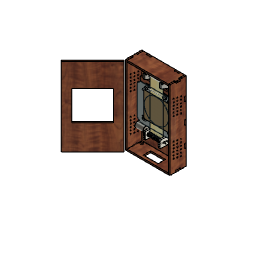
Target Holder v0 (Autodesk Fusion 360 design; units mm, degrees)
Autodesk Fusion 360 part; units mm, degrees
note: some values were not read from the file. Set by a fixed rule: which face or edge a step refers to.
(part 1 of 4)
sketch "Sketch8" plane through (0, 0, 0) normal (0, 1, 0) x (1, 0, 0)
  line L0 (-142.6941, 256.8986) -> (-422.6941, 256.8986)
  line L1 (-232.6941, -163.1014) -> (-332.6941, -163.1014)
  line L2 (-365.1941, -98.1014) -> (-200.1941, -98.1014)
  line L3 (-200.1941, -98.1014) -> (-200.1941, 66.8986)
  line L4 (-200.1941, 66.8986) -> (-365.1941, 66.8986)
  line L5 (-365.1941, 66.8986) -> (-365.1941, -98.1014)
  line L6 (-392.6941, -273.1014) -> (-362.6941, -273.1014)
  line L7 (-362.6941, -273.1014) -> (-362.6941, -263.1014)
  line L8 (-392.6941, -263.1014) -> (-392.6941, -273.1014)
  line L9 (-432.6941, -18.1014) -> (-422.6941, -18.1014)
  line L10 (-422.6941, 11.8986) -> (-432.6941, 11.8986)
  line L11 (-432.6941, 11.8986) -> (-432.6941, -18.1014)
  line L12 (-142.6941, -18.1014) -> (-132.6941, -18.1014)
  line L13 (-132.6941, -18.1014) -> (-132.6941, 11.8986)
  line L14 (-132.6941, 11.8986) -> (-142.6941, 11.8986)
  line L15 (-432.6941, -155.6014) -> (-422.6941, -155.6014)
  line L16 (-422.6941, -125.6014) -> (-432.6941, -125.6014)
  line L17 (-432.6941, -125.6014) -> (-432.6941, -155.6014)
  line L18 (-142.6941, 119.3986) -> (-132.6941, 119.3986)
  line L19 (-132.6941, 119.3986) -> (-132.6941, 149.3986)
  line L20 (-132.6941, 149.3986) -> (-142.6941, 149.3986)
  line L21 (-142.6941, -140.6014) -> (-132.6941, -140.6014)
  line L22 (-132.6941, -140.6014) -> (-132.6941, -110.6014)
  line L23 (-132.6941, -110.6014) -> (-142.6941, -110.6014)
  line L24 (-432.6941, 119.3986) -> (-422.6941, 119.3986)
  line L25 (-422.6941, 149.3986) -> (-432.6941, 149.3986)
  line L26 (-432.6941, 149.3986) -> (-432.6941, 119.3986)
  line L27 (-422.6941, -23.1014) -> (-422.6941, -120.6038)
  line L28 (-422.6941, -155.6014) -> (-422.6941, -263.1014)
  line L29 (-422.6941, 256.8986) -> (-422.6941, 154.3986)
  line L30 (-422.6941, 114.3986) -> (-422.6941, 16.8986)
  line L31 (-142.6941, 16.8986) -> (-142.6941, 114.3986)
  line L32 (-142.6941, 149.3986) -> (-142.6941, 256.8986)
  line L33 (-142.6941, -263.1014) -> (-142.6941, -145.6014)
  line L34 (-142.6941, -105.6014) -> (-142.6941, -23.1014)
  line L35 (-422.6941, -263.1014) -> (-397.6941, -263.1014)
  line L36 (-357.6941, -263.1014) -> (-332.6941, -263.1014)
  arc A0 (-422.6941, -160.6014) -> (-422.6941, -155.6014) centre (-422.6941, -158.1014) ccw
  arc A1 (-422.8505, -125.6014) -> (-422.6941, -120.6038) centre (-422.7723, -123.1026) ccw
  arc A2 (-422.6941, -23.1014) -> (-422.6941, -18.1014) centre (-422.6941, -20.6014) ccw
  arc A3 (-422.6941, 11.8986) -> (-422.6941, 16.8986) centre (-422.6941, 14.3986) ccw
  arc A4 (-142.6941, -18.1014) -> (-142.6941, -23.1014) centre (-142.6941, -20.6014) ccw
  arc A5 (-142.6941, 16.8986) -> (-142.6941, 11.8986) centre (-142.6941, 14.3986) ccw
  arc A6 (-142.6941, -140.6014) -> (-142.6941, -145.6014) centre (-142.6941, -143.1014) ccw
  arc A7 (-142.6941, -105.6014) -> (-142.6941, -110.6014) centre (-142.6941, -108.1014) ccw
  arc A8 (-392.6941, -263.1014) -> (-397.6941, -263.1014) centre (-395.1941, -263.1014) ccw
  arc A9 (-357.6941, -263.1014) -> (-362.6941, -263.1014) centre (-360.1941, -263.1014) ccw
  line L37 (-202.6941, -273.1014) -> (-172.6941, -273.1014)
  line L38 (-172.6941, -273.1014) -> (-172.6941, -263.1014)
  line L39 (-202.6941, -263.1014) -> (-202.6941, -273.1014)
  arc A10 (-202.6941, -263.1014) -> (-207.6941, -263.1014) centre (-205.1941, -263.1014) ccw
  line L40 (-232.6941, -263.1014) -> (-207.6941, -263.1014)
  line L41 (-167.6941, -263.1014) -> (-142.6941, -263.1014)
  arc A11 (-167.6941, -263.1014) -> (-172.6941, -263.1014) centre (-170.1941, -263.1014) ccw
  arc A12 (-422.6941, 114.3986) -> (-422.6941, 119.3986) centre (-422.6941, 116.8986) ccw
  arc A13 (-422.6941, 149.3986) -> (-422.6941, 154.3986) centre (-422.6941, 151.8986) ccw
  arc A14 (-142.6941, 119.3986) -> (-142.6941, 114.3986) centre (-142.6941, 116.8986) ccw
  arc A15 (-142.6941, 154.3986) -> (-142.6941, 149.3986) centre (-142.6941, 151.8986) ccw
  line L42 (-332.6941, -163.1014) -> (-232.6941, -163.1014)
  line L43 (-232.6941, -213.1014) -> (-332.6941, -213.1014)
  line L44 (-232.6941, -198.1014) -> (-232.6941, -200.1678)
  line L45 (-342.6941, -198.1014) -> (-332.6941, -198.1014)
  line L46 (-332.6941, -178.1014) -> (-342.6941, -178.1014)
  line L47 (-342.6941, -183.1014) -> (-342.6941, -193.1014)
  line L48 (-332.6941, -163.1014) -> (-332.6941, -178.1014)
  line L49 (-332.6941, -198.1014) -> (-332.6941, -263.1014)
  line L50 (-332.6941, -213.1014) -> (-332.6941, -198.1014)
  line L51 (-332.6941, -178.1014) -> (-332.6941, -163.1014)
  line L52 (-232.6941, -198.1014) -> (-222.6941, -198.1014)
  line L53 (-222.6941, -178.1014) -> (-232.6941, -178.1014)
  line L54 (-232.6941, -263.1014) -> (-232.6941, -198.1014)
  line L55 (-232.6941, -178.1014) -> (-232.6941, -163.1014)
  line L56 (-232.6941, -163.1014) -> (-232.6941, -178.1014)
  line L57 (-232.6941, -198.1014) -> (-232.6941, -213.1014)
  arc A16 (-222.6941, -198.1014) -> (-222.6941, -193.1014) centre (-222.6941, -195.6014) ccw
  arc A17 (-222.6941, -183.1014) -> (-222.6941, -178.1014) centre (-222.6941, -180.6014) ccw
  arc A18 (-342.6941, -193.1014) -> (-342.6941, -198.1014) centre (-342.6941, -195.6014) ccw
  arc A19 (-342.6941, -178.1014) -> (-342.6941, -183.1014) centre (-342.6941, -180.6014) ccw
  line L58 (-222.6941, -193.1014) -> (-222.6941, -183.1014)
  dimension "d24" = 280
  dimension "d25" = 520
  dimension "d26" = 100
  dimension "d27" = 100
  dimension "d28" = 165
  dimension "d29" = 165
  dimension "d36" = 30
  dimension "d37" = 10
  dimension "d40" = 10
  dimension "d41" = 30
  dimension "d42" = 10
  dimension "d43" = 30
  dimension "d44" = 10
  dimension "d45" = 30
  dimension "d46" = 10
  dimension "d47" = 30
  dimension "d48" = 10
  dimension "d49" = 30
  dimension "d50" = 10
  dimension "d51" = 30
  dimension "d52" = 5
  dimension "d53" = 5
  dimension "d54" = 5
  dimension "d55" = 5
  dimension "d56" = 5
  dimension "d57" = 5
  dimension "d58" = 5
  dimension "d59" = 5
  dimension "d60" = 5
  dimension "d61" = 5
  dimension "d63" = 30
  dimension "d64" = 10
  dimension "d65" = 5
  dimension "d66" = 5
  dimension "d67" = 5
  dimension "d68" = 5
  dimension "d69" = 5
  dimension "d70" = 5
  dimension "d73" = 50
  dimension "d76" = 10
  dimension "d77" = 20
  dimension "d78" = 10
  dimension "d79" = 20
  dimension "d80" = 5
  dimension "d81" = 5
  dimension "d82" = 5
  dimension "d84" = 5
  constraint horizontal L35
  constraint vertical L33
  constraint horizontal L0
  constraint vertical L29
  constraint vertical L54
  constraint horizontal L1
  constraint vertical L48
  constraint horizontal L2
  constraint vertical L3
  constraint horizontal L4
  constraint vertical L5
  constraint horizontal L6
  constraint vertical L7
  constraint vertical L8
  constraint horizontal L9
  constraint horizontal L10
  constraint vertical L11
  constraint horizontal L12
  constraint vertical L13
  constraint horizontal L14
  constraint horizontal L15
  constraint horizontal L16
  constraint vertical L17
  constraint horizontal L18
  constraint vertical L19
  constraint horizontal L20
  constraint horizontal L21
  constraint vertical L22
  constraint horizontal L23
  constraint collinear L31 L33
  constraint collinear L27 L29
  constraint horizontal L24
  constraint horizontal L25
  constraint vertical L26
  constraint collinear L27 L28
  constraint collinear L29 L30
  constraint collinear L31 L32
  constraint collinear L33 L34
  constraint collinear L35 L36
  constraint coincident L16.start A1
  constraint coincident L28 A0.start
  constraint coincident L16 A1.start
  constraint perpendicular L33 L40
  constraint horizontal L37
  constraint vertical L38
  constraint vertical L39
  constraint collinear L40 L41
  constraint coincident L32 A15.start
  constraint horizontal L42
  constraint vertical L56
  constraint horizontal L43
  constraint vertical L50
  constraint vertical L44
  constraint coincident L44.end L54
  constraint coincident L44.end L56
  constraint horizontal L45
  constraint horizontal L46
  constraint vertical L47
  constraint collinear L48 L49
  constraint collinear L50 L51
  constraint horizontal L52
  constraint horizontal L53
  constraint collinear L54 L55
  constraint collinear L56 L57
  constraint vertical L58
  measures "d24" distance of L28.end L33.start
  measures "d25" distance of L28.end L0.end
  measures "d26" distance of L36.end L40.start
  measures "d27" distance of L36.end L1.end
  measures "d28" distance of L2.start L2.end
  measures "d29" distance of L2.start L4.end
  measures "d36" distance of L6.start L6.end
  measures "d37" distance of L6.start L8.start
  measures "d40" distance of L9.start L9.end
  measures "d41" distance of L9.start L10.end
  measures "d42" distance of L12.start L12.end
  measures "d43" distance of L12.start L14.end
  measures "d44" distance of L15.start L15.end
  measures "d45" distance of L15.start L16.end
  measures "d46" distance of L18.start L18.end
  measures "d47" distance of L18.start L20.end
  measures "d48" distance of L21.start L21.end
  measures "d49" distance of L21.start L23.end
  measures "d50" distance of L24.start L24.end
  measures "d51" distance of L24.start L25.end
  measures "d52" diameter of A0
  measures "d53" diameter of A1
  measures "d54" diameter of A2
  measures "d55" diameter of A3
  measures "d56" diameter of A4
  measures "d57" diameter of A5
  measures "d58" diameter of A6
  measures "d59" diameter of A7
  measures "d60" diameter of A8
  measures "d61" diameter of A9
  measures "d63" distance of L37.start L37.end
  measures "d64" distance of L37.start L39.start
  measures "d65" diameter of A10
  measures "d66" diameter of A11
  measures "d67" diameter of A12
  measures "d68" diameter of A13
  measures "d69" diameter of A15
  measures "d70" diameter of A14
  measures "d73" distance of L1.end L43.end
  measures "d76" distance of L45.start L45.end
  measures "d77" distance of L45.start L46.end
  measures "d78" distance of L44.start L52.end
  measures "d79" distance of L44.start L53.end
  measures "d80" diameter of A17
  measures "d81" diameter of A16
  measures "d82" diameter of A19
  measures "d84" diameter of A18
sketch "Sketch9" plane through (0, 0, 0) normal (0, 1, 0) x (1, 0, 0)
extrude "Extrude1" add sketch "Sketch8" along normal blind 10 contours L0 L1 L6 L7 L8 L9 L10 L11 L12 L13 L14 L15 L16 L17 L18 L19 L20 L21 L22 L23 L24 L25 L26 L27 L28 L29 L30 L31 L32 L33 L34 L35 L36 A0 A1 A2 A3 A4 A5 A6 A7 A8 A9 L37 L38 L39 A10 L40 L41 A11 A12 A13 A14 A15 L42 L44 L45 L46 L47 L48 L49 L50 L51 L52 L53 L54 L55 L56 L57 A16 A17 A18 A19 L58 makes body 1
sketch "Sketch1" plane through (0, 0, 0) normal (1, 0, 0) x (0, 1, 0) in component "Side"
sketch "Sketch2" plane through (-142.6941, 0, 0) normal (1, 0, 0) x (0, 1, 0) in component "Side"
sketch "Sketch3" plane through (0, 0, 0) normal (0, -1, 0) x (1, 0, 0) in component "Side"
sketch "Sketch10" plane through (-142.6941, 0, 0) normal (1, 0, 0) x (0, 1, 0)
  line L0 (-100, -256.3488) -> (-100, 273.6512)
  line L1 (0, -119.3986) -> (10, -119.3986)
  line L2 (10, -149.3986) -> (0, -149.3986)
  line L3 (0, -144.3986) -> (0, -124.3986)
  line L4 (0, 140.6014) -> (10, 140.6014)
  line L5 (10, 110.6014) -> (0, 110.6014)
  line L6 (0, 110.6014) -> (0, 115.6014)
  line L7 (0, 18.1014) -> (10, 18.1014)
  line L8 (10, -11.8986) -> (0, -11.8986)
  line L9 (0, -6.8986) -> (0, 13.1014)
  line L10 (10, 273.6512) -> (10, 140.6014)
  arc A0 (0, 140.6014) -> (0, 135.6014) centre (0, 138.1014) ccw
  arc A1 (0, 115.6014) -> (0, 110.6014) centre (0, 113.1014) ccw
  line L11 (10, 110.6014) -> (10, 18.1014)
  arc A2 (0, -6.8986) -> (0, -11.8986) centre (0, -9.3986) ccw
  arc A3 (0, 18.1014) -> (0, 13.1014) centre (0, 15.6014) ccw
  arc A4 (0, -119.3986) -> (0, -124.3986) centre (0, -121.8986) ccw
  arc A5 (0, -144.3986) -> (0, -149.3986) centre (0, -146.8986) ccw
  line L12 (-30, 273.6512) -> (-30, 263.6512)
  line L13 (-35, 263.6512) -> (-55, 263.6512)
  line L14 (-60, 263.6512) -> (-60, 273.6512)
  line L15 (-100, 273.6512) -> (-60, 273.6512)
  line L16 (-30, 273.6512) -> (10, 273.6512)
  arc A6 (-60, 263.6512) -> (-55, 263.6512) centre (-57.5, 263.6512) ccw
  arc A7 (-35, 263.6512) -> (-30, 263.6512) centre (-32.5, 263.6512) ccw
  circle A8 centre (-75, 230) radius 4
  circle A9 centre (-55, 225) radius 4
  circle A10 centre (-35, 220) radius 4
  line L17 (-55, -246.3488) -> (-35, -246.3488)
  line L18 (-30, -246.3488) -> (-30, -256.3488)
  line L19 (-60, -256.3488) -> (-60, -246.3488)
  line L20 (10, -256.3488) -> (-30, -256.3488)
  line L21 (-60, -256.3488) -> (-100, -256.3488)
  arc A11 (-55, -246.3488) -> (-60, -246.3488) centre (-57.5, -246.3488) ccw
  arc A12 (-30, -246.3488) -> (-35, -246.3488) centre (-32.5, -246.3488) ccw
  line L22 (10, -11.8986) -> (10, -119.3986)
  line L23 (10, -149.3986) -> (10, -256.3488)
  line L24 (0, 135.6014) -> (0, 115.6014)
  point P0 (0, -256.8986)
  point P1 (0, -119.3986)
  point P2 (0, 140.6014)
  point P3 (0, 18.1014)
  point P4 (-75, 215)
  point P5 (-75, 200)
  point P6 (-75, 185)
  point P7 (-75, 170)
  point P8 (-75, 155)
  point P9 (-75, 140)
  point P10 (-75, 125)
  point P11 (-75, 110)
  point P12 (-75, 95)
  point P13 (-75, 80)
  point P14 (-75, 65)
  point P15 (-75, 50)
  point P16 (-75, 35)
  point P17 (-75, 20)
  point P18 (-75, 5)
  point P19 (-75, -10)
  point P20 (-75, -25)
  point P21 (-75, -40)
  point P22 (-75, -55)
  point P23 (-75, -70)
  point P24 (-75, -85)
  point P25 (-75, -100)
  point P26 (-75, -115)
  point P27 (-75, -130)
  point P28 (-75, -145)
  point P29 (-75, -160)
  point P30 (-75, -175)
  point P31 (-75, -190)
  point P32 (-75, -205)
  point P33 (-55, 210)
  point P34 (-55, 195)
  point P35 (-55, 180)
  point P36 (-55, 165)
  point P37 (-55, 150)
  point P38 (-55, 135)
  point P39 (-55, 120)
  point P40 (-55, 105)
  point P41 (-55, 90)
  point P42 (-55, 75)
  point P43 (-55, 60)
  point P44 (-55, 45)
  point P45 (-55, 30)
  point P46 (-55, 15)
  point P47 (-55, 0)
  point P48 (-55, -15)
  point P49 (-55, -30)
  point P50 (-55, -45)
  point P51 (-55, -60)
  point P52 (-55, -75)
  point P53 (-55, -90)
  point P54 (-55, -105)
  point P55 (-55, -120)
  point P56 (-55, -135)
  point P57 (-55, -150)
  point P58 (-55, -165)
  point P59 (-55, -180)
  point P60 (-55, -195)
  point P61 (-55, -210)
  point P62 (-35, 205)
  point P63 (-35, 190)
  point P64 (-35, 175)
  point P65 (-35, 160)
  point P66 (-35, 145)
  point P67 (-35, 130)
  point P68 (-35, 115)
  point P69 (-35, 100)
  point P70 (-35, 85)
  point P71 (-35, 70)
  point P72 (-35, 55)
  point P73 (-35, 40)
  point P74 (-35, 25)
  point P75 (-35, 10)
  point P76 (-35, -5)
  point P77 (-35, -20)
  point P78 (-35, -35)
  point P79 (-35, -50)
  point P80 (-35, -65)
  point P81 (-35, -80)
  point P82 (-35, -95)
  point P83 (-35, -110)
  point P84 (-35, -125)
  point P85 (-35, -140)
  point P86 (-35, -155)
  point P87 (-35, -170)
  point P88 (-35, -185)
  point P89 (-35, -200)
  point P90 (-35, -215)
  dimension "d92" = 10
  dimension "d93" = 30
  dimension "d94" = 10
  dimension "d95" = 30
  dimension "d96" = 10
  dimension "d97" = 30
  dimension "d99" = 5
  dimension "d100" = 5
  dimension "d101" = 5
  dimension "d102" = 5
  dimension "d103" = 5
  dimension "d104" = 5
  dimension "d107" = 30
  dimension "d108" = 10
  dimension "d109" = 5
  dimension "d110" = 5
  dimension "d113" = 8
  dimension "d116" = 15
  dimension "d117" = -15
  dimension "d120" = 8
  dimension "d122" = 8
  dimension "d129" = 0
  dimension "d130" = -15
  dimension "d131" = 30
  dimension "d132" = 10
  dimension "d133" = 5
  dimension "d134" = 5
  constraint vertical L10
  constraint horizontal L20
  constraint vertical L0
  constraint horizontal L1
  constraint horizontal L2
  constraint vertical L3
  constraint coincident P1 L1.start
  constraint horizontal L4
  constraint horizontal L5
  constraint vertical L6
  constraint coincident P2 L4.start
  constraint horizontal L7
  constraint horizontal L8
  constraint vertical L9
  constraint coincident P3 L7.start
  constraint coincident P2 A0
  constraint collinear L10 L11
  constraint collinear L11 L22
  constraint coincident P1 A4
  constraint perpendicular L10 L15
  constraint vertical L12
  constraint horizontal L13
  constraint vertical L14
  constraint collinear L15 L16
  constraint horizontal L17
  constraint vertical L18
  constraint vertical L19
  constraint collinear L20 L21
  constraint collinear L22 L23
  constraint parallel L6 L24
  measures "d92" distance of P1 L1.end
  measures "d93" distance of P1 L2.end
  measures "d94" distance of P2 L4.end
  measures "d95" distance of P2 L5.end
  measures "d96" distance of P3 L7.end
  measures "d97" distance of P3 L8.end
  measures "d99" diameter of A0
  measures "d100" diameter of A1
  measures "d101" diameter of A3
  measures "d102" diameter of A2
  measures "d103" diameter of A4
  measures "d104" diameter of A5
  measures "d107" distance of L14.end L12.start
  measures "d108" distance of L14.end L14.start
  measures "d109" diameter of A7
  measures "d110" diameter of A6
  measures "d113" diameter of A8
  measures "d120" diameter of A9
  measures "d122" diameter of A10
  measures "d131" distance of L19.end L18.start
  measures "d132" distance of L19.end L19.start
  measures "d133" diameter of A12
  measures "d134" diameter of A11
sketch "Sketch11" plane through (-142.6941, 0, 0) normal (1, 0, 0) x (0, 1, 0)
extrude "Extrude2" add sketch "Sketch10" along normal blind 10 separate body contours L0 L1 L2 L3 L4 L5 L7 L8 L9 L10 A0 A1 L11 A2 A3 A4 A5 L12 L13 L14 L15 L16 A6 A7 L17 L18 L19 L20 L21 A11 A12 L22 L23 L24 | L6 A1 | A8 | A9 | A10 makes body 2
sketch "Sketch12" plane through (-132.6941, 0, 0) normal (1, 0, 0) x (0, 1, 0)
  line L0 (0, 140.6014) -> (10, 140.6014)
  line L1 (10, 140.6014) -> (10, 273.6512)
  line L2 (10, 273.6512) -> (-30, 273.6512)
  line L3 (-30, 273.6512) -> (-30, 263.6512)
  arc A0 (-35, 263.6512) -> (-30, 263.6512) centre (-32.5, 263.6512) ccw
  line L4 (-35, 263.6512) -> (-55, 263.6512)
  arc A1 (-60, 263.6512) -> (-55, 263.6512) centre (-57.5, 263.6512) ccw
  line L5 (-60, 263.6512) -> (-60, 273.6512)
  line L6 (-60, 273.6512) -> (-100, 273.6512)
  line L7 (-100, 273.6512) -> (-100, -256.3488)
  line L8 (-100, -256.3488) -> (-60, -256.3488)
  line L9 (-60, -256.3488) -> (-60, -246.3488)
  arc A2 (-55, -246.3488) -> (-60, -246.3488) centre (-57.5, -246.3488) ccw
  line L10 (-55, -246.3488) -> (-35, -246.3488)
  arc A3 (-30, -246.3488) -> (-35, -246.3488) centre (-32.5, -246.3488) ccw
  line L11 (-30, -246.3488) -> (-30, -256.3488)
  line L12 (-30, -256.3488) -> (10, -256.3488)
  line L13 (10, -256.3488) -> (10, -149.3986)
  line L14 (10, -149.3986) -> (0, -149.3986)
  arc A4 (0, -144.3986) -> (0, -149.3986) centre (0, -146.8986) ccw
  line L15 (0, -144.3986) -> (0, -124.3986)
  arc A5 (0, -119.3986) -> (0, -124.3986) centre (0, -121.8986) ccw
  line L16 (0, -119.3986) -> (10, -119.3986)
  line L17 (10, -119.3986) -> (10, -11.8986)
  line L18 (10, -11.8986) -> (0, -11.8986)
  arc A6 (0, -6.8986) -> (0, -11.8986) centre (0, -9.3986) ccw
  line L19 (0, -6.8986) -> (0, 13.1014)
  arc A7 (0, 18.1014) -> (0, 13.1014) centre (0, 15.6014) ccw
  line L20 (0, 18.1014) -> (10, 18.1014)
  line L21 (10, 18.1014) -> (10, 110.6014)
  line L22 (10, 110.6014) -> (0, 110.6014)
  line L23 (0, 110.6014) -> (0, 135.6014)
  arc A8 (0, 140.6014) -> (0, 135.6014) centre (0, 138.1014) ccw
  arc A9 (0, 115.6014) -> (0, 110.6014) centre (0, 113.1014) ccw
  dimension "d137" = 5
  constraint coincident L23 A9.start
  measures "d137" diameter of A9
sketch "Sketch13" plane through (-132.6941, 0, 0) normal (1, 0, 0) x (0, 1, 0)
sketch "Sketch14" plane through (-132.6941, 0, 0) normal (1, 0, 0) x (0, 1, 0)
extrude "Extrude3" cut sketch "Sketch12" against normal blind 10 contours L23 A9 bodies 2
sketch "Sketch19" plane through (-132.6941, 0, 0) normal (1, 0, 0) x (0, 1, 0)
  arc A0 (0, 115.6014) -> (0, 110.6014) centre (0, 113.1014) ccw
  line L0 (0, 115.6014) -> (0, 135.6014)
  arc A1 (0, 140.6014) -> (0, 135.6014) centre (0, 138.1014) ccw
  line L1 (0, 140.6014) -> (10, 140.6014)
  line L2 (10, 140.6014) -> (10, 273.6512)
  line L3 (10, 273.6512) -> (-30, 273.6512)
  line L4 (-30, 273.6512) -> (-30, 263.6512)
  arc A2 (-35, 263.6512) -> (-30, 263.6512) centre (-32.5, 263.6512) ccw
  line L5 (-35, 263.6512) -> (-55, 263.6512)
  arc A3 (-60, 263.6512) -> (-55, 263.6512) centre (-57.5, 263.6512) ccw
  line L6 (-60, 263.6512) -> (-60, 273.6512)
  line L7 (-60, 273.6512) -> (-100, 273.6512)
  line L8 (-100, 273.6512) -> (-100, -256.3488)
  line L9 (-100, -256.3488) -> (-60, -256.3488)
  line L10 (-60, -256.3488) -> (-60, -246.3488)
  arc A4 (-55, -246.3488) -> (-60, -246.3488) centre (-57.5, -246.3488) ccw
  line L11 (-55, -246.3488) -> (-35, -246.3488)
  arc A5 (-30, -246.3488) -> (-35, -246.3488) centre (-32.5, -246.3488) ccw
  line L12 (-30, -246.3488) -> (-30, -256.3488)
  line L13 (-30, -256.3488) -> (10, -256.3488)
  line L14 (10, -256.3488) -> (10, -149.3986)
  line L15 (10, -149.3986) -> (0, -149.3986)
  arc A6 (0, -144.3986) -> (0, -149.3986) centre (0, -146.8986) ccw
  line L16 (0, -144.3986) -> (0, -124.3986)
  arc A7 (0, -119.3986) -> (0, -124.3986) centre (0, -121.8986) ccw
  line L17 (0, -119.3986) -> (10, -119.3986)
  line L18 (10, -119.3986) -> (10, -11.8986)
  line L19 (10, -11.8986) -> (0, -11.8986)
  arc A8 (0, -6.8986) -> (0, -11.8986) centre (0, -9.3986) ccw
  line L20 (0, -6.8986) -> (0, 13.1014)
  arc A9 (0, 18.1014) -> (0, 13.1014) centre (0, 15.6014) ccw
  line L21 (0, 18.1014) -> (10, 18.1014)
  line L22 (10, 18.1014) -> (10, 110.6014)
  line L23 (10, 110.6014) -> (0, 110.6014)
  line L24 (-100, -170) -> (-100, 180)
  circle A10 centre (-75, 180) radius 4
  circle A11 centre (-50, 175) radius 4
  circle A12 centre (-25, 170) radius 4
  circle A13 centre (-75, -170) radius 4
  circle A14 centre (-50, -175) radius 4
  circle A15 centre (-25, -180) radius 4
  dimension "d160" = 25
  dimension "d161" = 350
  dimension "d166" = 8
  dimension "d167" = 8
  dimension "d168" = 8
  dimension "d170" = 8
  dimension "d171" = 8
  dimension "d172" = 8
  constraint vertical L24
  measures "d160" distance of L24.end A10.centre
  measures "d161" distance of L24.end L24.start
  measures "d166" diameter of A10
  measures "d167" diameter of A11
  measures "d168" diameter of A12
  measures "d170" diameter of A13
  measures "d171" diameter of A14
  measures "d172" diameter of A15
extrude "Extrude5" cut sketch "Sketch19" against normal blind 10 contours A10 | A11 | A12 | A13 | A14 | A15 bodies 2
copy_body "CopyPasteBodies1" bodies 2 makes body 3
move_body "Move1" bodies 3 to x (1, 0, 0) y (0, 1, 0) z (0, 0, 1) at (-280, 0, 0)
move_body "Move2" bodies 3 to x (1, 0, 0) y (0, 1, 0) z (0, 0, 1) at (-10, 0, 0)
sketch "Sketch20" plane through (0, 0, 0) normal (0, -1, 0) x (1, 0, 0)
  line L0 (-365.1941, 98.1014) -> (-200.1941, 98.1014)
  line L1 (-200.1941, 98.1014) -> (-200.1941, -66.8986)
  line L2 (-200.1941, -66.8986) -> (-365.1941, -66.8986)
  line L3 (-365.1941, -66.8986) -> (-365.1941, 98.1014)
  line L4 (-142.6941, -104.3986) -> (-422.6941, -104.3986)
  line L5 (-422.6941, -104.3986) -> (-422.6941, 135.6014)
  line L6 (-422.6941, 135.6014) -> (-142.6941, 135.6014)
  line L7 (-142.6941, 135.6014) -> (-142.6941, -104.3986)
  point P0 (-200.1941, 98.1014)
  dimension "d175" = 165
  dimension "d176" = 165
  dimension "d177" = 280
  dimension "d178" = 240
  constraint horizontal L0
  constraint vertical L1
  constraint horizontal L2
  constraint vertical L3
  constraint coincident P0 L0.end
  constraint horizontal L4
  constraint vertical L5
  constraint horizontal L6
  constraint vertical L7
  measures "d175" distance of L0.start P0
  measures "d176" distance of L0.start L2.end
  measures "d177" distance of L4.start L4.end
  measures "d178" distance of L4.start L6.end
extrude "Extrude6" add sketch "Sketch20" along normal blind 10 separate body makes body 4
sketch "Sketch21" plane through (0, 0, 0) normal (0, -1, 0) x (1, 0, 0)
  line L0 (-142.6471, 155.6014) -> (-132.6471, 155.6014)
  line L1 (-132.6471, 155.6014) -> (-132.6471, 125.6014)
  line L2 (-132.6471, 125.6014) -> (-142.6471, 125.6014)
  line L3 (-142.6471, 125.6014) -> (-142.6471, 155.6014)
  circle A0 centre (-142.6471, 158.1014) radius 2.5
  circle A1 centre (-142.6471, 123.1014) radius 2.5
  point P0 (-432.6941, 155.6014)
  dimension "d181" = 10
  dimension "d182" = 30
  dimension "d183" = 5
  dimension "d184" = 5
  constraint horizontal L0
  constraint vertical L1
  constraint horizontal L2
  constraint vertical L3
  constraint coincident L0.start A0
  constraint coincident L2.end A1
  measures "d181" distance of L0.start L0.end
  measures "d182" distance of L0.start L2.end
  measures "d183" diameter of A0
  measures "d184" diameter of A1
extrude "Extrude7" cut sketch "Sketch21" against normal blind 10 contours A1 | A0 bodies 1
sketch "Sketch22" plane through (0, 0, 0) normal (0, -1, 0) x (1, 0, 0)
  line L0 (-142.6941, 155.5705) -> (-132.6941, 155.5705)
  line L1 (-132.6941, 155.5705) -> (-132.6941, 125.5705)
  line L2 (-132.6941, 125.5705) -> (-142.6941, 125.5705)
  line L3 (-142.6941, 125.5705) -> (-142.6941, 155.5705)
  line L4 (-142.6941, 145.6014) -> (-142.6941, 263.1014)
  dimension "d187" = 10
  dimension "d188" = 30
  constraint horizontal L0
  constraint vertical L1
  constraint horizontal L2
  constraint vertical L3
  constraint coincident L0.start L4
  measures "d187" distance of L0.start L0.end
  measures "d188" distance of L0.start L2.end
extrude "Extrude8" add sketch "Sketch22" against normal blind 10 bodies 1
sketch "Sketch23" plane through (0, 0, 0) normal (0, -1, 0) x (1, 0, 0)
  line L0 (-132.6941, 110.6014) -> (-142.6941, 110.6014)
  line L1 (-142.6941, 110.6014) -> (-142.6941, 125.6014)
  line L2 (-142.6941, 125.6014) -> (-132.6941, 125.6014)
  line L3 (-132.6941, 125.6014) -> (-132.6941, 110.6014)
  point P0 (-132.6941, 110.6014)
  dimension "d191" = 10
  dimension "d192" = 15
  constraint horizontal L0
  constraint vertical L1
  constraint horizontal L2
  constraint vertical L3
  constraint coincident P0 L0.start
  measures "d191" distance of P0 L0.end
  measures "d192" distance of P0 L2.end
extrude "Extrude9" cut sketch "Sketch23" against normal blind 10 bodies 1
sketch "Sketch24" plane through (0, 0, 0) normal (0, -1, 0) x (1, 0, 0)
  line L0 (-150, 150) -> (-137.9691, 150)
  line L1 (-137.9691, 150) -> (-137.9691, 134.9927)
  line L2 (-137.9691, 134.9927) -> (-150, 134.9927)
  line L3 (-150, 134.9927) -> (-150, 150)
  line L4 (-161.0971, 97.7239) -> (-142.6941, 97.7239)
  line L5 (-142.6941, 97.7239) -> (-142.6941, 120.6018)
  line L6 (-142.6941, 120.6018) -> (-161.0971, 120.6018)
  line L7 (-161.0971, 120.6018) -> (-161.0971, 97.7239)
  point P0 (-142.6941, 120.6018)
  constraint horizontal L0
  constraint vertical L1
  constraint horizontal L2
  constraint vertical L3
  constraint horizontal L4
  constraint vertical L5
  constraint horizontal L6
  constraint vertical L7
  constraint coincident P0 L5.end
extrude "Extrude10" add sketch "Sketch24" against normal blind 10 bodies 1
sketch "Sketch25" plane through (-132.6941, 0, 0) normal (1, 0, 0) x (0, 1, 0)
  circle A0 centre (-75, -170) radius 4
  circle A1 centre (-75, 180) radius 4
  circle A2 centre (-50, -175) radius 4
  circle A3 centre (-25, 170) radius 4
  circle A4 centre (-50, 175) radius 4
  circle A5 centre (-25, -180) radius 4
  arc A6 (0, 115.6014) -> (0, 110.6014) centre (0, 113.1014) ccw
  line L0 (0, 115.6014) -> (0, 135.6014)
  arc A7 (0, 140.6014) -> (0, 135.6014) centre (0, 138.1014) ccw
  line L1 (0, 140.6014) -> (10, 140.6014)
  line L2 (10, 140.6014) -> (10, 273.6512)
  line L3 (10, 273.6512) -> (-30, 273.6512)
  line L4 (-30, 273.6512) -> (-30, 263.6512)
  arc A8 (-35, 263.6512) -> (-30, 263.6512) centre (-32.5, 263.6512) ccw
  line L5 (-35, 263.6512) -> (-55, 263.6512)
  arc A9 (-60, 263.6512) -> (-55, 263.6512) centre (-57.5, 263.6512) ccw
  line L6 (-60, 263.6512) -> (-60, 273.6512)
  line L7 (-60, 273.6512) -> (-100, 273.6512)
  line L8 (-100, 273.6512) -> (-100, -256.3488)
  line L9 (-100, -256.3488) -> (-60, -256.3488)
  line L10 (-60, -256.3488) -> (-60, -246.3488)
  arc A10 (-55, -246.3488) -> (-60, -246.3488) centre (-57.5, -246.3488) ccw
  line L11 (-55, -246.3488) -> (-35, -246.3488)
  arc A11 (-30, -246.3488) -> (-35, -246.3488) centre (-32.5, -246.3488) ccw
  line L12 (-30, -246.3488) -> (-30, -256.3488)
  line L13 (-30, -256.3488) -> (10, -256.3488)
  line L14 (10, -256.3488) -> (10, -149.3986)
  line L15 (10, -149.3986) -> (0, -149.3986)
  arc A12 (0, -144.3986) -> (0, -149.3986) centre (0, -146.8986) ccw
  line L16 (0, -144.3986) -> (0, -124.3986)
  arc A13 (0, -119.3986) -> (0, -124.3986) centre (0, -121.8986) ccw
  line L17 (0, -119.3986) -> (10, -119.3986)
  line L18 (10, -119.3986) -> (10, -11.8986)
  line L19 (10, -11.8986) -> (0, -11.8986)
  arc A14 (0, -6.8986) -> (0, -11.8986) centre (0, -9.3986) ccw
  line L20 (0, -6.8986) -> (0, 13.1014)
  arc A15 (0, 18.1014) -> (0, 13.1014) centre (0, 15.6014) ccw
  line L21 (0, 18.1014) -> (10, 18.1014)
  line L22 (10, 18.1014) -> (10, 110.6014)
  line L23 (10, 110.6014) -> (0, 110.6014)
  line L24 (0, 155.6014) -> (10, 155.6014)
  line L25 (10, 155.6014) -> (10, 140.6014)
  line L26 (10, 140.6014) -> (0, 140.6014)
  line L27 (0, 140.6014) -> (0, 155.6014)
  circle A16 centre (0, 153.1014) radius 2.5
  dimension "d197" = 10
  dimension "d198" = 15
  dimension "d199" = 5
  constraint horizontal L24
  constraint vertical L25
  constraint horizontal L26
  constraint vertical L27
  constraint coincident L1.end L2.start
  constraint coincident L24.start A16
  measures "d197" distance of L24.start L24.end
  measures "d198" distance of L24.start A7.start
  measures "d199" diameter of A16
extrude "Extrude11" cut sketch "Sketch25" against normal blind 10 contours L1 L2 L24 L25 L26 L27 A16 | L27 A16 | L27 A16 bodies 2
sketch "Sketch26" plane through (-132.6941, 0, 0) normal (1, 0, 0) x (0, 1, 0)
  line L0 (0, 155.6014) -> (10, 155.6014)
  line L1 (10, 155.6014) -> (10, 273.6512)
  line L2 (10, 273.6512) -> (-30, 273.6512)
  line L3 (-30, 273.6512) -> (-30, 263.6512)
  arc A0 (-35, 263.6512) -> (-30, 263.6512) centre (-32.5, 263.6512) ccw
  line L4 (-35, 263.6512) -> (-55, 263.6512)
  arc A1 (-60, 263.6512) -> (-55, 263.6512) centre (-57.5, 263.6512) ccw
  line L5 (-60, 263.6512) -> (-60, 273.6512)
  line L6 (-60, 273.6512) -> (-100, 273.6512)
  line L7 (-100, 273.6512) -> (-100, -256.3488)
  line L8 (-100, -256.3488) -> (-60, -256.3488)
  line L9 (-60, -256.3488) -> (-60, -246.3488)
  arc A2 (-55, -246.3488) -> (-60, -246.3488) centre (-57.5, -246.3488) ccw
  line L10 (-55, -246.3488) -> (-35, -246.3488)
  arc A3 (-30, -246.3488) -> (-35, -246.3488) centre (-32.5, -246.3488) ccw
  line L11 (-30, -246.3488) -> (-30, -256.3488)
  line L12 (-30, -256.3488) -> (10, -256.3488)
  line L13 (10, -256.3488) -> (10, -149.3986)
  line L14 (10, -149.3986) -> (0, -149.3986)
  arc A4 (0, -144.3986) -> (0, -149.3986) centre (0, -146.8986) ccw
  line L15 (0, -144.3986) -> (0, -124.3986)
  arc A5 (0, -119.3986) -> (0, -124.3986) centre (0, -121.8986) ccw
  line L16 (0, -119.3986) -> (10, -119.3986)
  line L17 (10, -119.3986) -> (10, -11.8986)
  line L18 (10, -11.8986) -> (0, -11.8986)
  arc A6 (0, -6.8986) -> (0, -11.8986) centre (0, -9.3986) ccw
  line L19 (0, -6.8986) -> (0, 13.1014)
  arc A7 (0, 18.1014) -> (0, 13.1014) centre (0, 15.6014) ccw
  line L20 (0, 18.1014) -> (10, 18.1014)
  line L21 (10, 18.1014) -> (10, 110.6014)
  line L22 (10, 110.6014) -> (0, 110.6014)
  arc A8 (0, 115.6014) -> (0, 110.6014) centre (0, 113.1014) ccw
  line L23 (0, 115.6014) -> (0, 135.6014)
  arc A9 (0, 140.6014) -> (0, 135.6014) centre (0, 138.1014) ccw
  line L24 (0, 140.6014) -> (0, 150.6014)
  arc A10 (0, 155.6014) -> (0, 150.6014) centre (0, 153.1014) ccw
  circle A11 centre (-75, -170) radius 4
  circle A12 centre (-75, 180) radius 4
  circle A13 centre (-50, -175) radius 4
  circle A14 centre (-25, 170) radius 4
  circle A15 centre (-50, 175) radius 4
  circle A16 centre (-25, -180) radius 4
  line L25 (10, 110.6014) -> (-5, 110.6014)
  line L26 (-5, 110.6014) -> (-5, 125.6014)
  line L27 (-5, 125.6014) -> (10, 125.6014)
  line L28 (10, 125.6014) -> (10, 110.6014)
  line L29 (0, 135.6014) -> (-10, 135.6014)
  line L30 (-10, 135.6014) -> (-10, 145.6014)
  line L31 (-10, 145.6014) -> (0, 145.6014)
  line L32 (0, 145.6014) -> (0, 135.6014)
  dimension "d202" = 15
  dimension "d203" = 15
  dimension "d204" = 10
  dimension "d205" = 10
  constraint horizontal L25
  constraint vertical L26
  constraint horizontal L27
  constraint vertical L28
  constraint coincident L21.end L22.start
  constraint horizontal L29
  constraint vertical L30
  constraint horizontal L31
  constraint vertical L32
  constraint coincident L23.end A9.end
  measures "d202" distance of L21.end L25.end
  measures "d203" distance of L21.end L27.end
  measures "d204" distance of L23.end L29.end
  measures "d205" distance of L23.end L31.end
extrude "Extrude12" add sketch "Sketch26" against normal blind 10 contours A9 L24 L29 L30 L31 L32 | L22 A8 L23 L25 L27 L28 bodies 2
sketch "Sketch27" plane through (-132.6941, 0, 0) normal (1, 0, 0) x (0, 1, 0)
  circle A0 centre (-25, -180) radius 4
  circle A1 centre (-50, 175) radius 4
  circle A2 centre (-25, 170) radius 4
  circle A3 centre (-50, -175) radius 4
  circle A4 centre (-75, 180) radius 4
  circle A5 centre (-75, -170) radius 4
  arc A6 (0, 140.6014) -> (0, 135.6014) centre (0, 138.1014) ccw
  line L0 (0, 140.6014) -> (0, 150.6014)
  arc A7 (0, 155.6014) -> (0, 150.6014) centre (0, 153.1014) ccw
  line L1 (0, 155.6014) -> (10, 155.6014)
  line L2 (10, 155.6014) -> (10, 273.6512)
  line L3 (10, 273.6512) -> (-30, 273.6512)
  line L4 (-30, 273.6512) -> (-30, 263.6512)
  arc A8 (-35, 263.6512) -> (-30, 263.6512) centre (-32.5, 263.6512) ccw
  line L5 (-35, 263.6512) -> (-55, 263.6512)
  arc A9 (-60, 263.6512) -> (-55, 263.6512) centre (-57.5, 263.6512) ccw
  line L6 (-60, 263.6512) -> (-60, 273.6512)
  line L7 (-60, 273.6512) -> (-100, 273.6512)
  line L8 (-100, 273.6512) -> (-100, -256.3488)
  line L9 (-100, -256.3488) -> (-60, -256.3488)
  line L10 (-60, -256.3488) -> (-60, -246.3488)
  arc A10 (-55, -246.3488) -> (-60, -246.3488) centre (-57.5, -246.3488) ccw
  line L11 (-55, -246.3488) -> (-35, -246.3488)
  arc A11 (-30, -246.3488) -> (-35, -246.3488) centre (-32.5, -246.3488) ccw
  line L12 (-30, -246.3488) -> (-30, -256.3488)
  line L13 (-30, -256.3488) -> (10, -256.3488)
  line L14 (10, -256.3488) -> (10, -149.3986)
  line L15 (10, -149.3986) -> (0, -149.3986)
  arc A12 (0, -144.3986) -> (0, -149.3986) centre (0, -146.8986) ccw
  line L16 (0, -144.3986) -> (0, -124.3986)
  arc A13 (0, -119.3986) -> (0, -124.3986) centre (0, -121.8986) ccw
  line L17 (0, -119.3986) -> (10, -119.3986)
  line L18 (10, -119.3986) -> (10, -11.8986)
  line L19 (10, -11.8986) -> (0, -11.8986)
  arc A14 (0, -6.8986) -> (0, -11.8986) centre (0, -9.3986) ccw
  line L20 (0, -6.8986) -> (0, 13.1014)
  arc A15 (0, 18.1014) -> (0, 13.1014) centre (0, 15.6014) ccw
  line L21 (0, 18.1014) -> (10, 18.1014)
  line L22 (10, 18.1014) -> (10, 125.6014)
  line L23 (10, 125.6014) -> (0, 125.6014)
  line L24 (0, 125.6014) -> (0, 135.6014)
  circle A16 centre (0, 128.1014) radius 2.5
  dimension "d208" = 5
  constraint coincident L23.end A16
  measures "d208" diameter of A16
extrude "Extrude13" cut sketch "Sketch27" against normal blind 10 contours L24 A16 | L24 A16 bodies 2
sketch "Sketch28" plane through (-132.6941, 0, 0) normal (1, 0, 0) x (0, 1, 0)
  arc A0 (0, 130.6014) -> (0, 125.6014) centre (0, 128.1014) ccw
  line L0 (0, 130.6014) -> (0, 135.6014)
  arc A1 (0, 140.6014) -> (0, 135.6014) centre (0, 138.1014) ccw
  line L1 (0, 140.6014) -> (0, 150.6014)
  arc A2 (0, 155.6014) -> (0, 150.6014) centre (0, 153.1014) ccw
  line L2 (0, 155.6014) -> (10, 155.6014)
  line L3 (10, 155.6014) -> (10, 273.6512)
  line L4 (10, 273.6512) -> (-30, 273.6512)
  line L5 (-30, 273.6512) -> (-30, 263.6512)
  arc A3 (-35, 263.6512) -> (-30, 263.6512) centre (-32.5, 263.6512) ccw
  line L6 (-35, 263.6512) -> (-55, 263.6512)
  arc A4 (-60, 263.6512) -> (-55, 263.6512) centre (-57.5, 263.6512) ccw
  line L7 (-60, 263.6512) -> (-60, 273.6512)
  line L8 (-60, 273.6512) -> (-100, 273.6512)
  line L9 (-100, 273.6512) -> (-100, -256.3488)
  line L10 (-100, -256.3488) -> (-60, -256.3488)
  line L11 (-60, -256.3488) -> (-60, -246.3488)
  arc A5 (-55, -246.3488) -> (-60, -246.3488) centre (-57.5, -246.3488) ccw
  line L12 (-55, -246.3488) -> (-35, -246.3488)
  arc A6 (-30, -246.3488) -> (-35, -246.3488) centre (-32.5, -246.3488) ccw
  line L13 (-30, -246.3488) -> (-30, -256.3488)
  line L14 (-30, -256.3488) -> (10, -256.3488)
  line L15 (10, -256.3488) -> (10, -149.3986)
  line L16 (10, -149.3986) -> (0, -149.3986)
  arc A7 (0, -144.3986) -> (0, -149.3986) centre (0, -146.8986) ccw
  line L17 (0, -144.3986) -> (0, -124.3986)
  arc A8 (0, -119.3986) -> (0, -124.3986) centre (0, -121.8986) ccw
  line L18 (0, -119.3986) -> (10, -119.3986)
  line L19 (10, -119.3986) -> (10, -11.8986)
  line L20 (10, -11.8986) -> (0, -11.8986)
  arc A9 (0, -6.8986) -> (0, -11.8986) centre (0, -9.3986) ccw
  line L21 (0, -6.8986) -> (0, 13.1014)
  arc A10 (0, 18.1014) -> (0, 13.1014) centre (0, 15.6014) ccw
  line L22 (0, 18.1014) -> (10, 18.1014)
  line L23 (10, 18.1014) -> (10, 125.6014)
  line L24 (10, 125.6014) -> (0, 125.6014)
  circle A11 centre (-75, -170) radius 4
  circle A12 centre (-75, 180) radius 4
  circle A13 centre (-50, -175) radius 4
  circle A14 centre (-25, 170) radius 4
  circle A15 centre (-50, 175) radius 4
  circle A16 centre (-25, -180) radius 4
  line L25 (0, 135.6014) -> (-10.5923, 135.6014)
  line L26 (-10.5923, 135.6014) -> (-10.5923, 145.6014)
  line L27 (-10.5923, 145.6014) -> (0, 145.6014)
  line L28 (0, 145.6014) -> (0, 135.6014)
  dimension "d211" = 10.5923
  dimension "d212" = 10
  constraint horizontal L25
  constraint vertical L26
  constraint horizontal L27
  constraint vertical L28
  constraint coincident L0.end A1.end
  measures "d211" distance of L0.end L25.end
  measures "d212" distance of L0.end L27.end
extrude "Extrude14" add sketch "Sketch28" against normal blind 10 contours A1 L1 L25 L26 L27 L28 bodies 2
sketch "Sketch29" plane through (-132.6941, 0, 0) normal (1, 0, 0) x (0, 1, 0)
  circle A0 centre (-25, -180) radius 4
  circle A1 centre (-50, 175) radius 4
  circle A2 centre (-25, 170) radius 4
  circle A3 centre (-50, -175) radius 4
  circle A4 centre (-75, 180) radius 4
  circle A5 centre (-75, -170) radius 4
  arc A6 (0, 140.6014) -> (0, 135.6014) centre (0, 138.1014) ccw
  line L0 (0, 140.6014) -> (0, 150.6014)
  arc A7 (0, 155.6014) -> (0, 150.6014) centre (0, 153.1014) ccw
  line L1 (0, 155.6014) -> (10, 155.6014)
  line L2 (10, 155.6014) -> (10, 273.6512)
  line L3 (10, 273.6512) -> (-30, 273.6512)
  line L4 (-30, 273.6512) -> (-30, 263.6512)
  arc A8 (-35, 263.6512) -> (-30, 263.6512) centre (-32.5, 263.6512) ccw
  line L5 (-35, 263.6512) -> (-55, 263.6512)
  arc A9 (-60, 263.6512) -> (-55, 263.6512) centre (-57.5, 263.6512) ccw
  line L6 (-60, 263.6512) -> (-60, 273.6512)
  line L7 (-60, 273.6512) -> (-100, 273.6512)
  line L8 (-100, 273.6512) -> (-100, -256.3488)
  line L9 (-100, -256.3488) -> (-60, -256.3488)
  line L10 (-60, -256.3488) -> (-60, -246.3488)
  arc A10 (-55, -246.3488) -> (-60, -246.3488) centre (-57.5, -246.3488) ccw
  line L11 (-55, -246.3488) -> (-35, -246.3488)
  arc A11 (-30, -246.3488) -> (-35, -246.3488) centre (-32.5, -246.3488) ccw
  line L12 (-30, -246.3488) -> (-30, -256.3488)
  line L13 (-30, -256.3488) -> (10, -256.3488)
  line L14 (10, -256.3488) -> (10, -149.3986)
  line L15 (10, -149.3986) -> (0, -149.3986)
  arc A12 (0, -144.3986) -> (0, -149.3986) centre (0, -146.8986) ccw
  line L16 (0, -144.3986) -> (0, -124.3986)
  arc A13 (0, -119.3986) -> (0, -124.3986) centre (0, -121.8986) ccw
  line L17 (0, -119.3986) -> (10, -119.3986)
  line L18 (10, -119.3986) -> (10, -11.8986)
  line L19 (10, -11.8986) -> (0, -11.8986)
  arc A14 (0, -6.8986) -> (0, -11.8986) centre (0, -9.3986) ccw
  line L20 (0, -6.8986) -> (0, 13.1014)
  arc A15 (0, 18.1014) -> (0, 13.1014) centre (0, 15.6014) ccw
  line L21 (0, 18.1014) -> (10, 18.1014)
  line L22 (10, 18.1014) -> (10, 125.6014)
  line L23 (10, 125.6014) -> (0, 125.6014)
  arc A16 (0, 130.6014) -> (0, 125.6014) centre (0, 128.1014) ccw
  line L24 (0, 130.6014) -> (0, 135.6014)
  line L25 (-10, 145.6014) -> (0, 145.6014)
  line L26 (0, 145.6014) -> (0, 135.6014)
  line L27 (0, 135.6014) -> (-10, 135.6014)
  line L28 (-10, 135.6014) -> (-10, 145.6014)
  dimension "d215" = 10
  dimension "d216" = 10
  constraint horizontal L25
  constraint vertical L26
  constraint horizontal L27
  constraint vertical L28
  constraint coincident A6.end L24.end
  measures "d215" distance of L25.start L25.end
  measures "d216" distance of L25.start L27.end
sketch "Sketch36" plane through (-432.6941, 0, 0) normal (-1, 0, 0) x (0, -1, 0)
  circle A0 centre (75, -170) radius 4
  circle A1 centre (75, 180) radius 4
  circle A2 centre (50, -175) radius 4
  circle A3 centre (25, 170) radius 4
  circle A4 centre (50, 175) radius 4
  circle A5 centre (25, -180) radius 4
  arc A6 (0, 110.6014) -> (0, 115.6014) centre (0, 113.1014) ccw
  line L0 (0, 110.6014) -> (-10, 110.6014)
  line L1 (-10, 110.6014) -> (-10, 18.1014)
  line L2 (-10, 18.1014) -> (0, 18.1014)
  arc A7 (0, 13.1014) -> (0, 18.1014) centre (0, 15.6014) ccw
  line L3 (0, 13.1014) -> (0, -6.8986)
  arc A8 (0, -11.8986) -> (0, -6.8986) centre (0, -9.3986) ccw
  line L4 (0, -11.8986) -> (-10, -11.8986)
  line L5 (-10, -11.8986) -> (-10, -119.3986)
  line L6 (-10, -119.3986) -> (0, -119.3986)
  arc A9 (0, -124.3986) -> (0, -119.3986) centre (0, -121.8986) ccw
  line L7 (0, -124.3986) -> (0, -144.3986)
  arc A10 (0, -149.3986) -> (0, -144.3986) centre (0, -146.8986) ccw
  line L8 (0, -149.3986) -> (-10, -149.3986)
  line L9 (-10, -149.3986) -> (-10, -256.3488)
  line L10 (-10, -256.3488) -> (30, -256.3488)
  line L11 (30, -256.3488) -> (30, -246.3488)
  arc A11 (35, -246.3488) -> (30, -246.3488) centre (32.5, -246.3488) ccw
  line L12 (35, -246.3488) -> (55, -246.3488)
  arc A12 (60, -246.3488) -> (55, -246.3488) centre (57.5, -246.3488) ccw
  line L13 (60, -246.3488) -> (60, -256.3488)
  line L14 (60, -256.3488) -> (100, -256.3488)
  line L15 (100, -256.3488) -> (100, 273.6512)
  line L16 (100, 273.6512) -> (60, 273.6512)
  line L17 (60, 273.6512) -> (60, 263.6512)
  arc A13 (55, 263.6512) -> (60, 263.6512) centre (57.5, 263.6512) ccw
  line L18 (55, 263.6512) -> (35, 263.6512)
  arc A14 (30, 263.6512) -> (35, 263.6512) centre (32.5, 263.6512) ccw
  line L19 (30, 263.6512) -> (30, 273.6512)
  line L20 (30, 273.6512) -> (-10, 273.6512)
  line L21 (-10, 273.6512) -> (-10, 140.6014)
  line L22 (-10, 140.6014) -> (0, 140.6014)
  arc A15 (0, 135.6014) -> (0, 140.6014) centre (0, 138.1014) ccw
  line L23 (0, 135.6014) -> (0, 115.6014)
  line L24 (0, 155.6014) -> (-10, 155.6014)
  line L25 (-10, 155.6014) -> (-10, 125.6014)
  line L26 (-10, 125.6014) -> (0, 125.6014)
  line L27 (0, 125.6014) -> (0, 155.6014)
  circle A16 centre (0, 153.1014) radius 2.5
  point P0 (0, 155.6014)
  dimension "d229" = 10
  dimension "d230" = 30
  dimension "d231" = 5
  constraint horizontal L24
  constraint vertical L25
  constraint horizontal L26
  constraint vertical L27
  constraint coincident P0 L24.start
  constraint coincident P0 A16
  measures "d229" distance of P0 L24.end
  measures "d230" distance of P0 L26.end
  measures "d231" diameter of A16
extrude "Extrude17" cut sketch "Sketch36" against normal blind 10 contours L21 L22 L24 L25 L27 A16 | L27 A16 | L27 A16 bodies 3
sketch "Sketch37" plane through (-432.6941, 0, 0) normal (-1, 0, 0) x (0, -1, 0)
  line L0 (0, 150.6014) -> (0, 140.6014)
  arc A0 (0, 135.6014) -> (0, 140.6014) centre (0, 138.1014) ccw
  line L1 (0, 135.6014) -> (0, 115.6014)
  arc A1 (0, 110.6014) -> (0, 115.6014) centre (0, 113.1014) ccw
  line L2 (0, 110.6014) -> (-10, 110.6014)
  line L3 (-10, 110.6014) -> (-10, 18.1014)
  line L4 (-10, 18.1014) -> (0, 18.1014)
  arc A2 (0, 13.1014) -> (0, 18.1014) centre (0, 15.6014) ccw
  line L5 (0, 13.1014) -> (0, -6.8986)
  arc A3 (0, -11.8986) -> (0, -6.8986) centre (0, -9.3986) ccw
  line L6 (0, -11.8986) -> (-10, -11.8986)
  line L7 (-10, -11.8986) -> (-10, -119.3986)
  line L8 (-10, -119.3986) -> (0, -119.3986)
  arc A4 (0, -124.3986) -> (0, -119.3986) centre (0, -121.8986) ccw
  line L9 (0, -124.3986) -> (0, -144.3986)
  arc A5 (0, -149.3986) -> (0, -144.3986) centre (0, -146.8986) ccw
  line L10 (0, -149.3986) -> (-10, -149.3986)
  line L11 (-10, -149.3986) -> (-10, -256.3488)
  line L12 (-10, -256.3488) -> (30, -256.3488)
  line L13 (30, -256.3488) -> (30, -246.3488)
  arc A6 (35, -246.3488) -> (30, -246.3488) centre (32.5, -246.3488) ccw
  line L14 (35, -246.3488) -> (55, -246.3488)
  arc A7 (60, -246.3488) -> (55, -246.3488) centre (57.5, -246.3488) ccw
  line L15 (60, -246.3488) -> (60, -256.3488)
  line L16 (60, -256.3488) -> (100, -256.3488)
  line L17 (100, -256.3488) -> (100, 273.6512)
  line L18 (100, 273.6512) -> (60, 273.6512)
  line L19 (60, 273.6512) -> (60, 263.6512)
  arc A8 (55, 263.6512) -> (60, 263.6512) centre (57.5, 263.6512) ccw
  line L20 (55, 263.6512) -> (35, 263.6512)
  arc A9 (30, 263.6512) -> (35, 263.6512) centre (32.5, 263.6512) ccw
  line L21 (30, 263.6512) -> (30, 273.6512)
  line L22 (30, 273.6512) -> (-10, 273.6512)
  line L23 (-10, 273.6512) -> (-10, 155.6014)
  line L24 (-10, 155.6014) -> (0, 155.6014)
  arc A10 (0, 150.6014) -> (0, 155.6014) centre (0, 153.1014) ccw
  circle A11 centre (75, -170) radius 4
  circle A12 centre (75, 180) radius 4
  circle A13 centre (50, -175) radius 4
  circle A14 centre (25, 170) radius 4
  circle A15 centre (50, 175) radius 4
  circle A16 centre (25, -180) radius 4
  line L25 (-10, 110.6014) -> (5, 110.6014)
  line L26 (5, 110.6014) -> (5, 125.6014)
  line L27 (5, 125.6014) -> (-10, 125.6014)
  line L28 (-10, 125.6014) -> (-10, 110.6014)
  dimension "d234" = 15
  dimension "d235" = 15
  constraint horizontal L25
  constraint vertical L26
  constraint horizontal L27
  constraint vertical L28
  constraint coincident L2.end L3.start
  measures "d234" distance of L2.end L25.end
  measures "d235" distance of L2.end L27.end
extrude "Extrude18" add sketch "Sketch37" against normal blind 10 contours L1 A1 L2 L25 L27 L28 bodies 3
sketch "Sketch38" plane through (-432.6941, 0, 0) normal (-1, 0, 0) x (0, -1, 0)
  line L0 (0, 150.6014) -> (0, 140.6014)
  arc A0 (0, 135.6014) -> (0, 140.6014) centre (0, 138.1014) ccw
  line L1 (0, 135.6014) -> (0, 125.6014)
  line L2 (0, 125.6014) -> (-10, 125.6014)
  line L3 (-10, 125.6014) -> (-10, 18.1014)
  line L4 (-10, 18.1014) -> (0, 18.1014)
  arc A1 (0, 13.1014) -> (0, 18.1014) centre (0, 15.6014) ccw
  line L5 (0, 13.1014) -> (0, -6.8986)
  arc A2 (0, -11.8986) -> (0, -6.8986) centre (0, -9.3986) ccw
  line L6 (0, -11.8986) -> (-10, -11.8986)
  line L7 (-10, -11.8986) -> (-10, -119.3986)
  line L8 (-10, -119.3986) -> (0, -119.3986)
  arc A3 (0, -124.3986) -> (0, -119.3986) centre (0, -121.8986) ccw
  line L9 (0, -124.3986) -> (0, -144.3986)
  arc A4 (0, -149.3986) -> (0, -144.3986) centre (0, -146.8986) ccw
  line L10 (0, -149.3986) -> (-10, -149.3986)
  line L11 (-10, -149.3986) -> (-10, -256.3488)
  line L12 (-10, -256.3488) -> (30, -256.3488)
  line L13 (30, -256.3488) -> (30, -246.3488)
  arc A5 (35, -246.3488) -> (30, -246.3488) centre (32.5, -246.3488) ccw
  line L14 (35, -246.3488) -> (55, -246.3488)
  arc A6 (60, -246.3488) -> (55, -246.3488) centre (57.5, -246.3488) ccw
  line L15 (60, -246.3488) -> (60, -256.3488)
  line L16 (60, -256.3488) -> (100, -256.3488)
  line L17 (100, -256.3488) -> (100, 273.6512)
  line L18 (100, 273.6512) -> (60, 273.6512)
  line L19 (60, 273.6512) -> (60, 263.6512)
  arc A7 (55, 263.6512) -> (60, 263.6512) centre (57.5, 263.6512) ccw
  line L20 (55, 263.6512) -> (35, 263.6512)
  arc A8 (30, 263.6512) -> (35, 263.6512) centre (32.5, 263.6512) ccw
  line L21 (30, 263.6512) -> (30, 273.6512)
  line L22 (30, 273.6512) -> (-10, 273.6512)
  line L23 (-10, 273.6512) -> (-10, 155.6014)
  line L24 (-10, 155.6014) -> (0, 155.6014)
  arc A9 (0, 150.6014) -> (0, 155.6014) centre (0, 153.1014) ccw
  circle A10 centre (75, -170) radius 4
  circle A11 centre (75, 180) radius 4
  circle A12 centre (50, -175) radius 4
  circle A13 centre (25, 170) radius 4
  circle A14 centre (50, 175) radius 4
  circle A15 centre (25, -180) radius 4
  circle A16 centre (0, 128.1014) radius 2.5
  dimension "d238" = 5
  constraint coincident L1.end A16
  measures "d238" diameter of A16
extrude "Extrude19" cut sketch "Sketch38" against normal blind 10 contours L1 A16 picked at (1.3934, 128.5519) bodies 3